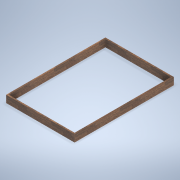
# Autodesk Inventor part: solar panels holder 2
Saved by Autodesk Inventor 2020 (Build 240168000, 168)
## iProperties
Created: 2020-06-26
Part Number: solar panels holder 2
Material: Generic
Document SubType Name: Modeling
Designer: Abbas
Density: 1 g/cm^3
Appearance: Default
Author: Abbas
Autodesk Inventor part; units mm, degrees
ref_plane "YZ Plane" through (0, 0, 0) normal (1, 0, 0) x (0, 1, 0)
ref_plane "XZ Plane" through (0, 0, 0) normal (0, 1, 0) x (-1, 0, 0)
ref_plane "XY Plane" through (0, 0, 0) normal (0, 0, 1) x (1, 0, 0)
sketch "Sketch1" plane through (0, 0, 0) normal (0, 1, 0) x (-1, 0, 0)
  line L0 (478.912, 694) -> (-478.912, 694)
  line L1 (-478.912, 694) -> (-478.912, -694)
  line L2 (-478.912, -694) -> (478.912, -694)
  line L3 (478.912, -694) -> (478.912, 694)
  line L4 (478.912, 694) -> (-478.912, -694) construction
  line L5 (-478.912, 694) -> (478.912, -694) construction
  line L6 (458.912, 674) -> (-458.912, 674)
  line L7 (-458.912, 674) -> (-458.912, -674)
  line L8 (-458.912, -674) -> (458.912, -674)
  line L9 (458.912, -674) -> (458.912, 674)
  line L10 (458.912, 674) -> (-458.912, -674) construction
  line L11 (-458.912, 674) -> (458.912, -674) construction
  point P0 (0, 0)
  point P1 (458.912, 0)
  point P2 (-448.912, 0)
  point P3 (-458.912, 0)
  point P4 (0, 674)
  point P5 (0, -674)
  dimension "d0" = 957.824
  dimension "d1" = 1388
  dimension "d2" = 917.824
  dimension "d3" = 1348
  constraints: 24 end point, 8 midpoint, 4 parallel, 2 horizontal, 2 perpendicular
  measures "d0" distance of L2.end L1.end
  measures "d1" distance of L1.end L0.end
  measures "d2" distance of L8.end L7.end
  measures "d3" distance of L7.end L6.end
extrude "Extrusion7" add sketch "Sketch1" along normal blind 100
sketch "Sketch2" plane through (478.912, 0, 694) normal (1, 0, 0) x (0, 0, -1)
  line L0 (0, 0) -> (0, 100) projected
  line L1 (0, 100) -> (1388, 100) projected
  point P0 (694, 0)
  point P1 (40, 75)
  dimension "d40" = 40
  dimension "d41" = 25
  measures "d40" distance from line of L0 point (40, 75)
  measures "d41" distance from line of L1 point (40, 75)
hole "Hole1" at (478.912, 75, 654) direction (-1, 0, 0) diameter 8 end through all
sketch "Sketch3" plane through (478.912, 0, 694) normal (1, 0, 0) x (0, 0, -1)
  line L0 (0, 0) -> (0, 100) projected
  line L1 (0, 0) -> (1388, 0) projected
  point P0 (694, 0)
  point P1 (40, 25)
  dimension "d42" = 40
  dimension "d43" = 25
  measures "d42" distance from line of L0 point (40, 25)
  measures "d43" distance from line of L1 point (40, 25)
hole "Hole2" at (478.912, 25, 654) direction (-1, 0, 0) diameter 8 end through all
sketch "Sketch4" plane through (478.912, 0, 694) normal (1, 0, 0) x (0, 0, -1)
  line L0 (1388, 0) -> (1388, 100) projected
  line L1 (0, 100) -> (1388, 100) projected
  point P0 (694, 0)
  point P1 (1348, 75)
  dimension "d58" = 40
  dimension "d59" = 25
  measures "d58" distance from line of L0 point (1348, 75)
  measures "d59" distance from line of L1 point (1348, 75)
hole "Hole3" at (478.912, 75, -654) direction (-1, 0, 0) diameter 8 end through all
sketch "Sketch5" plane through (478.912, 0, 694) normal (1, 0, 0) x (0, 0, -1)
  line L0 (1388, 0) -> (1388, 100) projected
  line L1 (0, 0) -> (1388, 0) projected
  point P0 (694, 0)
  point P1 (1348, 25)
  dimension "d60" = 40
  dimension "d61" = 25
  measures "d60" distance from line of L0 point (1348, 25)
  measures "d61" distance from line of L1 point (1348, 25)
hole "Hole4" at (478.912, 25, -654) direction (-1, 0, 0) diameter 8 end through all
sketch "Sketch6" plane through (-478.912, 0, 694) normal (0, 0, 1) x (1, 0, 0)
  line L0 (0, 100) -> (957.824, 100) projected
  line L1 (957.824, 0) -> (957.824, 100) projected
  line L2 (0, 0) -> (957.824, 0) projected
  point P0 (478.912, 0)
  point P1 (917.824, 75)
  point P2 (917.824, 25)
  dimension "d69" = 25
  dimension "d70" = 40
  dimension "d71" = 40
  dimension "d72" = 25
  measures "d69" distance from line of L0 point (917.824, 75)
  measures "d70" distance from line of L1 point (917.824, 75)
  measures "d71" distance from line of L1 point (917.824, 25)
  measures "d72" distance from line of L2 point (917.824, 25)
hole "Hole5" at (438.912, 75, 694) at (438.912, 25, 694) direction (0, 0, -1) diameter 8 end through all
sketch "Sketch7" plane through (-478.912, 0, 694) normal (0, 0, 1) x (1, 0, 0)
  line L0 (0, 0) -> (0, 100) projected
  line L1 (0, 100) -> (957.824, 100) projected
  point P0 (478.912, 0)
  point P1 (40, 75)
  dimension "d87" = 40
  dimension "d88" = 25
  measures "d87" distance from line of L0 point (40, 75)
  measures "d88" distance from line of L1 point (40, 75)
hole "Hole6" at (-438.912, 75, 694) direction (0, 0, -1) diameter 8 end through all
sketch "Sketch8" plane through (-478.912, 0, 694) normal (0, 0, 1) x (1, 0, 0)
  line L0 (0, 0) -> (0, 100) projected
  line L1 (0, 0) -> (957.824, 0) projected
  point P0 (478.912, 0)
  point P1 (40, 25)
  dimension "d89" = 40
  dimension "d90" = 25
  measures "d89" distance from line of L0 point (40, 25)
  measures "d90" distance from line of L1 point (40, 25)
hole "Hole7" at (-438.912, 25, 694) direction (0, 0, -1) diameter 8 end through all
body "Solid2"
